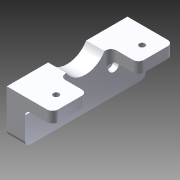
# Autodesk Inventor part: x-end right-side T
Saved by Autodesk Inventor 2015 SP1 (Build 190203100, 203)
## iProperties
Created: 2015-01-04
Part Number: x-end right-side T
Material: ABS Plastic
Document SubType Name: Modeling
Designer: Luna
Mass: 16.7904 g
Surface Area: 47.04 cm^2
Volume: 15.84 cm^3
Density: 1.06 g/cm^3
Appearance: Smooth - White
Author: Luna
Autodesk Inventor part; units mm, degrees
ref_plane "YZ Plane" through (0, 0, 0) normal (1, 0, 0) x (0, 1, 0)
ref_plane "XZ Plane" through (0, 0, 0) normal (0, 1, 0) x (-1, 0, 0)
ref_plane "XY Plane" through (0, 0, 0) normal (0, 0, 1) x (1, 0, 0)
sketch "Sketch1" plane through (0, 0, 0) normal (0, 0, 1) x (1, 0, 0)
  line L0 (-5, 33) -> (5, 33)
  line L1 (5, 33) -> (5, -33)
  line L2 (5, -33) -> (-5, -33)
  line L3 (-5, -33) -> (-5, 33)
  point P0 (0, 0)
  point P1 (5, 0)
  point P2 (0, 33)
  dimension "d0" = 10
  dimension "d1" = 66
  constraints: 8 end point, 2 midpoint, 2 parallel, 1 horizontal, 1 horizontal alignment, 1 perpendicular, 1 vertical alignment
  measures "d0" distance of L1.end L2.end
  measures "d1" distance of L0.end L1.end
extrude "Extrusion1" add sketch "Sketch1" along normal blind 24
fillet "Fillet1" radius 3 2 edges at (0, 33, 0) (0, -33, 0)
sketch "Sketch2" plane through (5, -33, 24) normal (1, 0, 0) x (0, 0, -1)
  arc A0 (21, 0) -> (24, 3) centre (21, 3) ccw projected
  line L0 (24, 63) -> (24, 3) projected
  arc A1 (24, 63) -> (21, 66) centre (21, 63) ccw projected
  line L1 (21, 66) -> (0, 66) projected
  line L2 (0, 0) -> (0, 66) projected
  line L3 (21, 0) -> (0, 0) projected
  line L4 (0, 66) -> (6, 66)
  line L5 (6, 66) -> (6, 47)
  line L6 (6, 47) -> (0, 47)
  line L7 (0, 47) -> (0, 66)
  line L8 (0, 0) -> (6, 0)
  line L9 (6, 0) -> (6, 19)
  line L10 (6, 19) -> (0, 19)
  line L11 (0, 19) -> (0, 0)
  point P0 (24, 33)
  point P1 (0, 56.5)
  point P2 (3, 66)
  dimension "d5" = 6
  dimension "d6" = 19
  dimension "d7" = 6
  dimension "d8" = 19
  constraints: 16 end point, 4 parallel, 2 horizontal, 2 midpoint, 2 perpendicular, 1 horizontal alignment, 1 vertical alignment
  measures "d5" distance of L5.end L6.end
  measures "d6" distance of L4.end L5.end
  measures "d7" distance of L10.end L9.end
  measures "d8" distance of L9.end L8.end
extrude "Extrusion2" add sketch "Sketch2" along normal blind 15 contours L3 L2 L10 L9 | L5 L6 L2 L1
sketch "Sketch5" plane through (5, -30, 0) normal (1, 0, 0) x (0, 0, -1)
  circle A0 centre (-14.5, 45.5) radius 1.5 projected
  circle A1 centre (-14.5, 14.5) radius 1.5 projected
  point P0 (0, 30)
hole "Hole2" at (5, 15.5, 14.5) at (5, -15.5, 14.5) direction (-1, 0, 0) diameter 3.2 end through all counterbore diameter 6 counterbore depth 3
sketch "Sketch6" plane through (5, 14, 18) normal (0, 0, -1) x (-1, 0, 0)
  circle A0 centre (-7.5, 9.5) radius 1.6 projected
  circle A1 centre (-7.5, -37.5) radius 1.6 projected
  point P0 (5, -14)
hole "Hole3" at (12.5, 23.5, 18) at (12.5, -23.5, 18) direction (0, 0, 1) diameter 3.2 end through all
sketch "Sketch7" plane through (5, 14, 18) normal (0, 0, -1) x (-1, 0, 0)
  circle A0 centre (-7.5, 9.5) radius 1.6 projected
  circle A1 centre (-7.5, -37.5) radius 1.6 projected
  line L0 (-4.2668, 9.5) -> (-5.8834, 6.7)
  line L1 (-5.8834, 6.7) -> (-9.1166, 6.7)
  line L2 (-9.1166, 6.7) -> (-10.7332, 9.5)
  line L3 (-10.7332, 9.5) -> (-9.1166, 12.3)
  line L4 (-9.1166, 12.3) -> (-5.8834, 12.3)
  line L5 (-5.8834, 12.3) -> (-4.2668, 9.5)
  line L6 (-5.8834, -40.3) -> (-9.1166, -40.3)
  line L7 (-9.1166, -40.3) -> (-10.7332, -37.5)
  line L8 (-10.7332, -37.5) -> (-9.1166, -34.7)
  line L9 (-9.1166, -34.7) -> (-5.8834, -34.7)
  line L10 (-5.8834, -34.7) -> (-4.2668, -37.5)
  line L11 (-4.2668, -37.5) -> (-5.8834, -40.3)
  line L12 (-15, 0) -> (-15, 19) projected
  line L13 (-15, -47) -> (-15, -28) projected
  point P0 (5, -14)
  point P1 (-15, -37.5)
  point P2 (-15, 9.5)
  dimension "d40" = 5.6
  dimension "d41" = 5.6
  constraints: 24 end point, 4 coincident, 2 horizontal alignment, 2 midpoint, 26 other
  measures "d40" distance between parallel lines of L1 L4
  measures "d41" distance between parallel lines of L6 L9
extrude "Extrusion4" cut sketch "Sketch7" against normal blind 3
fillet "Fillet4" radius 3 8 edges at (20, 33, 21) (20, -14, 21) (20, 14, 21) (20, -33, 21) (5, -23.5, 18) (5, 23.5, 18) (5, 14, 21) (5, -14, 21)
sketch "Sketch8" plane through (-5, -33, 24) normal (-1, 0, 0) x (0, 0, 1)
  circle A0 centre (6, 33) radius 11 projected
  circle A1 centre (6, 33) radius 12
  point P0 (-24, 33)
  dimension "d45" = 1
  constraints: 1 centre point
  measures "d45" radial gap between concentric circles of A0 A1
extrude "Extrusion5" cut sketch "Sketch8" against normal up to surface (10 mm away) contours A0 | A1
body "Solid1"
